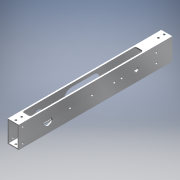
# Autodesk Inventor part: SideExtrusion
Saved by Autodesk Inventor 2019.4 (Build 234330000, 330)
## iProperties
Created: 2019-12-31
Part Number: SideExtrusion
Material: Aluminum 6061
Document SubType Name: Modeling
Designer: Mark
Mass: 418.792 g
Surface Area: 1108.63 cm^2
Volume: 155.108 cm^3
Density: 2.7 g/cm^3
Appearance: Aluminum - Flat
Author: Mark
Autodesk Inventor part; units mm, degrees
ref_plane "YZ Plane" through (0, 0, 0) normal (1, 0, 0) x (0, 1, 0)
ref_plane "XZ Plane" through (0, 0, 0) normal (0, 1, 0) x (-1, 0, 0)
ref_plane "XY Plane" through (0, 0, 0) normal (0, 0, 1) x (1, 0, 0)
sketch "Sketch1" plane through (0, 0, 0) normal (0, 0, 1) x (1, 0, 0)
  line L0 (-15, -30) -> (15, -30)
  line L1 (15, -30) -> (15, 30)
  line L2 (15, 30) -> (-15, 30)
  line L3 (-15, 30) -> (-15, -30)
  line L4 (-15, -30) -> (15, 30) construction
  line L5 (15, -30) -> (-15, 30) construction
  line L6 (-12, -27) -> (12, -27)
  line L7 (12, -27) -> (12, 27)
  line L8 (12, 27) -> (-12, 27)
  line L9 (-12, 27) -> (-12, -27)
  line L10 (-12, -27) -> (12, 27) construction
  line L11 (12, -27) -> (-12, 27) construction
  point P0 (0, 0)
  dimension "d0" = 30
  dimension "d1" = 60
  dimension "d2" = 24
  dimension "d3" = 54
  constraints: 24 end point, 4 midpoint, 4 parallel, 2 horizontal, 2 perpendicular
  measures "d0" distance of L2.end L1.end
  measures "d1" distance of L1.end L0.end
  measures "d2" distance of L8.end L7.end
  measures "d3" distance of L7.end L6.end
extrude "Extrusion1" add sketch "Sketch1" along normal blind 385
sketch "Sketch2" plane through (15, -30, 0) normal (1, 0, 0) x (0, 0, -1)
  circle A0 centre (-63.02, 30) radius 6
  line L0 (0, 60) -> (-385, 60) projected
  line L1 (0, 0) -> (0, 60) projected
  circle A1 centre (-304.72, 30) radius 12
  circle A2 centre (-183.87, 30) radius 2.75
  line L2 (0, 0) -> (-385, 0) projected
  circle A3 centre (-123.445, 30) radius 2.75
  circle A4 centre (-244.295, 30) radius 2.75
  circle A5 centre (-373.5, 50) radius 2.1
  circle A6 centre (-373.5, 10) radius 2.1
  line L3 (-385, 60) -> (-385, 0) projected
  line L4 (-213.87, 30) -> (-153.87, 30) construction
  line L5 (-213.87, 10) -> (-153.87, 10)
  line L6 (-153.87, 50) -> (-213.87, 50)
  arc A7 (-213.87, 50) -> (-213.87, 10) centre (-213.87, 30) ccw
  arc A8 (-153.87, 10) -> (-153.87, 50) centre (-153.87, 30) ccw
  point P0 (0, 30)
  point P1 (-183.87, 30)
  dimension "d6" = 12
  dimension "d7" = 30
  dimension "PulleyHole" = 63.02
  dimension "d18" = 24
  dimension "d19" = 30
  dimension "d20" = 241.7
  dimension "d30" = 5.5
  dimension "d31" = 30
  dimension "d32" = 120.85
  dimension "d33" = 5.5
  dimension "d34" = 5.5
  dimension "d35" = 30
  dimension "d36" = 30
  dimension "d37" = 60.425
  dimension "d38" = 60.425
  dimension "d39" = 4.2
  dimension "d40" = 4.2
  dimension "d41" = 10
  dimension "d42" = 11.5
  dimension "d43" = 10
  dimension "d44" = 11.5
  dimension "d56" = 40
  dimension "d57" = 30.425
  dimension "d59" = 60
  dimension "d60" = 10
  constraints: 9 centre point, 8 end point, 4 point on circle, 4 tangent, 1 horizontal, 1 midpoint, 1 parallel
  measures "d6" diameter of A0
  measures "d7" distance from line of L0 A0.centre
  measures "PulleyHole" distance from line of L1 A0.centre
  measures "d18" diameter of A1
  measures "d19" distance from line of L0 A1.centre
  measures "d20" distance of A0.centre A1.centre
  measures "d30" diameter of A2
  measures "d31" distance from line of L2 A2.centre
  measures "d32" distance of A1.centre A2.centre
  measures "d33" diameter of A3
  measures "d34" diameter of A4
  measures "d35" distance from line of L0 A4.centre
  measures "d36" distance from line of L0 A3.centre
  measures "d37" distance of A2.centre A3.centre
  measures "d38" distance of A2.centre A4.centre
  measures "d39" diameter of A5
  measures "d40" diameter of A6
  measures "d41" distance from line of L2 A6.centre
  measures "d42" distance from line of L3 A6.centre
  measures "d43" distance from line of L0 A5.centre
  measures "d44" distance from line of L3 A5.centre
  measures "d56" diameter of A8
  measures "d57" distance of A4.centre L4.start
  measures "d59" distance of L6.start L6.end
  measures "d60" distance between parallel lines of L2 L5
extrude "Extrusion2" cut sketch "Sketch2" against normal blind 30 contours A0 | A1 | A2 | A3 | A4 | A5 | A6
sketch "Sketch4" plane through (-15, 30, 0) normal (0, 1, 0) x (1, 0, 0)
  circle A0 centre (15, -63.02) radius 7.5 construction
  line L0 (0, 0) -> (0, -385) projected
  line L1 (30, 0) -> (0, 0) projected
  line L2 (26, -259.72) -> (4, -259.72)
  line L3 (4, -259.72) -> (4, -349.72)
  line L4 (4, -349.72) -> (26, -349.72)
  line L5 (26, -349.72) -> (26, -259.72)
  line L6 (26, -259.72) -> (4, -349.72) construction
  line L7 (4, -259.72) -> (26, -349.72) construction
  line L8 (4, -259.72) -> (26, -259.72)
  line L9 (26, -259.72) -> (26, -39.72)
  line L10 (26, -39.72) -> (4, -39.72)
  line L11 (4, -39.72) -> (4, -259.72)
  point P0 (15, 0)
  point P1 (15, -304.72)
  dimension "d13" = 15
  dimension "d14" = 15
  dimension "d15" = 63.02
  dimension "d23" = 22
  dimension "d24" = 15
  dimension "d25" = 90
  dimension "d26" = 241.7
  dimension "d28" = 22
  dimension "d29" = 220
  constraints: 20 end point, 4 parallel, 2 horizontal, 2 midpoint, 2 perpendicular, 1 centre point
  measures "d13" diameter of A0
  measures "d14" distance from line of L0 A0.centre
  measures "d15" distance from line of L1 A0.centre
  measures "d23" distance of L4.end L3.end
  measures "d24" distance from line of L0 point (15, -304.72)
  measures "d25" distance between parallel lines of L2 L4
  measures "d26" distance of A0.centre point (15, -304.72)
  measures "d28" distance of L10.end L9.end
  measures "d29" distance of L9.end L8.end
extrude "Extrusion4" cut sketch "Sketch4" against normal blind 87.25
sketch "Sketch5" plane through (-15, -30, 0) normal (-1, 0, 0) x (0, 0, 1)
  arc A0 (96.02, 56) -> (88.02, 60) centre (88.02, 50) ccw projected
  line L0 (88.02, 60) -> (30, 60) projected
  arc A1 (30, 60) -> (30, 0) centre (30, 30) ccw projected
  line L1 (30, 0) -> (63.02, 0) projected
  arc A2 (63.02, 0) -> (78.02, 4.0192) centre (63.02, 30) ccw projected
  line L2 (78.02, 4.0192) -> (108.02, 21.3397) projected
  arc A3 (108.02, 21.3397) -> (111.02, 36) centre (103.02, 30) ccw projected
  line L3 (111.02, 36) -> (96.02, 56) projected
  circle A4 centre (30, 30) radius 9.75 projected
  circle A5 centre (63.02, 30) radius 9.5 projected
  circle A6 centre (88.02, 55) radius 2.2 projected
  circle A7 centre (30, 4.6) radius 2.2 projected
  circle A8 centre (8.003, 17.3) radius 2.2 projected
  circle A9 centre (8.003, 42.7) radius 2.2 projected
  circle A10 centre (30, 55.4) radius 2.2 projected
  circle A11 centre (103.02, 30) radius 2.75 projected
  point P0 (0, 30)
extrude "Extrusion5" cut sketch "Sketch5" against normal blind 30 contours A8 | A9 | A11
fillet "Fillet1" radius 5 8 edges at (-11, -28.5, 349.72) (11, 28.5, 349.72) (11, -28.5, 349.72) (-11, 28.5, 349.72) (11, 28.5, 39.72) (-11, 28.5, 39.72) (-11, -28.5, 39.72) (11, -28.5, 39.72)
sketch "Sketch6" plane through (0, 0, 0) normal (0, 0, -1) x (-1, 0, 0)
  line L0 (12, 27) -> (12, -27) projected
  line L1 (12, -27) -> (-12, -27) projected
  line L2 (-12, -27) -> (-12, 27) projected
  line L3 (-12, 27) -> (12, 27) projected
  line L4 (15, -30) -> (-15, -30) projected
  line L5 (15, 30) -> (15, -30) projected
  line L6 (-15, 30) -> (15, 30) projected
  line L7 (-15, -30) -> (-15, 30) projected
  point P0 (0, 0)
extrude "Extrusion6" add sketch "Sketch6" along normal blind 35
sketch "Sketch8" plane through (-15, -30, 385) normal (-1, 0, 0) x (0, 0, 1)
  line L0 (-231.13, 30) -> (-171.13, 30) construction
  line L1 (-231.13, 10) -> (-171.13, 10)
  line L2 (-171.13, 50) -> (-231.13, 50)
  arc A0 (-231.13, 50) -> (-231.13, 10) centre (-231.13, 30) ccw
  arc A1 (-171.13, 10) -> (-171.13, 50) centre (-171.13, 30) ccw
  line L3 (-231.13, 30) -> (-171.13, 30) construction
  line L4 (0, 0) -> (-420, 0) projected
  circle A2 centre (-261.555, 30) radius 2.75 projected
  point P0 (-385, 30)
  point P1 (-201.13, 30)
  dimension "d61" = 60
  dimension "d62" = 0
  dimension "d63" = 40
  dimension "d64" = 10
  dimension "d65" = 30.425
  constraints: 10 end point, 4 point on circle, 4 tangent, 2 centre point, 2 horizontal, 1 collinear, 1 midpoint, 1 parallel
  measures "d61" distance of L0.start L0.end
  measures "d62" distance between parallel lines of L0 L3
  measures "d63" diameter of A1
  measures "d64" distance between parallel lines of L4 L1
  measures "d65" distance of A2.centre L0.start
extrude "Extrusion8" cut sketch "Sketch8" against normal blind 10 contours A0 L2 A1 L1
sketch "Sketch9" plane through (-15, 30, 385) normal (0, 1, 0) x (1, 0, 0)
  circle A0 centre (15, 413) radius 2.75
  circle A1 centre (15, 397) radius 2.75
  line L0 (0, 420) -> (0, 0) projected
  line L1 (0, 420) -> (30, 420) projected
  circle A2 centre (15, 7) radius 2.75
  circle A3 centre (15, 23) radius 2.75
  line L2 (30, 0) -> (0, 0) projected
  point P0 (15, 385)
  dimension "d68" = 5.5
  dimension "d69" = 5.5
  dimension "d70" = 15
  dimension "d71" = 15
  dimension "d72" = 7
  dimension "d73" = 16
  dimension "d74" = 5.5
  dimension "d75" = 5.5
  dimension "d76" = 15
  dimension "d77" = 15
  dimension "d78" = 7
  dimension "d79" = 16
  constraints: 4 centre point
  measures "d68" diameter of A0
  measures "d69" diameter of A1
  measures "d70" distance from line of L0 A0.centre
  measures "d71" distance from line of L0 A1.centre
  measures "d72" distance from line of L1 A0.centre
  measures "d73" distance of A0.centre A1.centre
  measures "d74" diameter of A2
  measures "d75" diameter of A3
  measures "d76" distance from line of L0 A3.centre
  measures "d77" distance from line of L0 A2.centre
  measures "d78" distance from line of L2 A2.centre
  measures "d79" distance of A2.centre A3.centre
extrude "Extrusion9" cut sketch "Sketch9" against normal up to surface (60 mm away)
equation "\"d15\" = PulleyHole"
body "Solid1"
